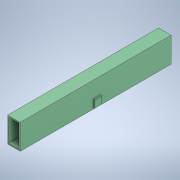
# Autodesk Inventor part: PerfilH34
Saved by Autodesk Inventor 2021 (Build 250183000, 183)
## iProperties
Created: 2021-06-11
Part Number: PerfilH34
Material: Generic
Document SubType Name: Modeling
Designer: lcper
Density: 1 g/cm^3
Appearance: Default
Author: lcper
Autodesk Inventor part; units mm, degrees
ref_plane "YZ Plane" through (0, 0, 0) normal (1, 0, 0) x (0, 1, 0)
ref_plane "XZ Plane" through (0, 0, 0) normal (0, 1, 0) x (-1, 0, 0)
ref_plane "XY Plane" through (0, 0, 0) normal (0, 0, 1) x (1, 0, 0)
sketch "Sketch1" plane through (0, 0, 0) normal (0, 0, 1) x (1, 0, 0)
  line L0 (-9.4777, 15.0257) -> (40.5223, 15.0257)
  line L1 (40.5223, 15.0257) -> (40.5223, -84.9743)
  line L2 (40.5223, -84.9743) -> (-9.4777, -84.9743)
  line L3 (-9.4777, -84.9743) -> (-9.4777, 15.0257)
  line L4 (35.5223, 10.0257) -> (-4.4777, 10.0257)
  line L5 (-4.4777, 10.0257) -> (-4.4777, -79.9743)
  line L6 (-4.4777, -79.9743) -> (35.5223, -79.9743)
  line L7 (35.5223, -79.9743) -> (35.5223, 10.0257)
  point P0 (0, 0)
  point P1 (0, 0)
  dimension "d0" = 50
  dimension "d1" = 100
  dimension "d2" = 5
  dimension "d3" = 90
  dimension "d4" = 5
  dimension "d5" = 40
  constraints: 16 end point, 4 parallel, 2 horizontal, 2 perpendicular
  measures "d0" distance of L1.end L2.end
  measures "d1" distance of L0.end L1.end
  measures "d2" distance between parallel lines of L4 L0
  measures "d3" distance of L6.end L4.start
  measures "d4" distance between parallel lines of L1 L7
  measures "d5" distance of L5.end L6.end
extrude "Extrusion1" add sketch "Sketch1" along normal blind 600
sketch "Sketch2" plane through (40.5223, 465.0257, 325) normal (1, 0, 0) x (0, 0, -1)
  line L0 (15, -545) -> (45, -545)
  line L1 (45, -545) -> (45, -515)
  line L2 (45, -515) -> (15, -515)
  line L3 (15, -515) -> (15, -545)
  line L4 (59.7557, 330.4367) -> (-23.1236, 330.4367)
  line L5 (325, -550) -> (-275, -550) projected
  line L6 (325, -550) -> (325, -450) projected
  point P0 (-7.4135, 330.4367)
  dimension "d14" = 30
  dimension "d15" = 30
  dimension "d16" = 5
  dimension "d17" = 280
  constraints: 10 end point, 2 parallel, 1 horizontal, 1 perpendicular
  measures "d14" distance of L1.end L2.end
  measures "d15" distance of L0.end L1.end
  measures "d16" distance between parallel lines of L5 L0
  measures "d17" distance between parallel lines of L6 L1
extrude "Extrusion2" add sketch "Sketch2" along normal blind 5
body "Solid1"
